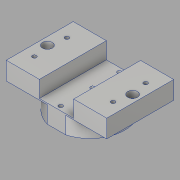
# Autodesk Inventor part: PocketNC_Vise_Backing_Plate
Saved by Autodesk Inventor 2017 (Build 210142000, 142)
## iProperties
Created: 2018-06-05
Part Number: PocketNC_Vise_Backing_Plate
Material: Aluminum 6061
Document SubType Name: Modeling
Designer: Jarrett
Density: 2.7 g/cm^3
Appearance: Aluminum - Flat
Author: Jarrett
Autodesk Inventor part; units mm, degrees
ref_plane "YZ Plane" through (0, 0, 0) normal (1, 0, 0) x (0, 1, 0)
ref_plane "XZ Plane" through (0, 0, 0) normal (0, 1, 0) x (-1, 0, 0)
ref_plane "XY Plane" through (0, 0, 0) normal (0, 0, 1) x (1, 0, 0)
sketch "Sketch1" plane through (0, 0, 0) normal (0, 1, 0) x (-1, 0, 0)
  line L0 (37.5, -25) -> (-37.5, -25) construction
  line L1 (-37.5, -25) -> (-37.5, 25) construction
  line L2 (-37.5, 25) -> (37.5, 25) construction
  line L3 (37.5, 25) -> (37.5, -25) construction
  arc A0 (6.8822, -25) -> (6.8822, 25) centre (0, 0) ccw
  arc A1 (-6.8822, 25) -> (-6.8822, -25) centre (0, 0) ccw
  line L4 (6.8822, -25) -> (-6.8822, -25)
  line L5 (-6.8822, 25) -> (6.8822, 25)
  dimension "d4" = 50
  dimension "d5" = 75
  constraints: 12 end point, 4 point on circle, 4 point on line, 2 centre point, 2 collinear, 1 coincident, 1 perpendicular, 1 vertical
  measures "d4" distance of L0.end L1.end
  measures "d5" distance of L1.end L2.end
extrude "Extrusion1" add sketch "Sketch1" along normal blind 12.65
sketch "Sketch2" plane through (0, 12.65, 0) normal (0, 1, 0) x (1, 0, 0)
  line L0 (-37.5, 25) -> (37.5, 25) construction
  line L1 (-37.5, -25) -> (-37.5, 25) construction
  line L2 (37.5, 25) -> (37.5, -25) construction
  line L3 (37.5, -25) -> (-37.5, -25) construction
  line L4 (-37.5, 25) -> (37.5, 25)
  line L5 (37.5, -25) -> (37.5, 25)
  line L6 (37.5, -25) -> (-37.5, -25)
  line L7 (-37.5, -25) -> (-37.5, 25)
  point P0 (0, 0)
  constraints: 8 end point, 2 collinear, 1 horizontal, 1 perpendicular
extrude "Extrusion2" add sketch "Sketch2" along normal blind 1
sketch "Sketch3" plane through (0, 13.65, 0) normal (0, 1, 0) x (1, 0, 0)
  line L0 (37.5, -25) -> (6.8822, -25) projected
  line L1 (12.8, -25) -> (12.8, 25)
  line L2 (12.8, 25) -> (37.5, 25)
  line L3 (37.5, -25) -> (37.5, 25) projected
  line L4 (37.5, 25) -> (37.5, -25)
  line L5 (37.5, -25) -> (12.8, -25)
  line L6 (-12.8, -25) -> (-12.8, 25)
  line L7 (-37.5, 25) -> (-37.5, -25) projected
  line L8 (-12.8, 25) -> (-37.5, 25)
  line L9 (-37.5, 25) -> (-37.5, -25)
  line L10 (-37.5, -25) -> (-12.8, -25)
  point P0 (0, 0)
  dimension "d12" = 25.6
  dimension "d13" = 24.7
  dimension "d14" = 24.7
  constraints: 16 end point, 4 perpendicular, 2 collinear, 2 point on line, 1 vertical
  measures "d12" distance between parallel lines of L1 L6
  measures "d13" distance of L6.end L7.start
  measures "d14" distance of L1.end L2.end
extrude "Extrusion3" add sketch "Sketch3" along normal blind 12.4 contours L10 L7 L8 L6
extrude "Extrusion4" add sketch "Sketch3" along normal blind 12.45 contours L0 L1 L2 L3
sketch "Sketch4" plane through (0, 13.65, 0) normal (0, 1, 0) x (1, 0, 0)
  circle A0 centre (0, 21.91) radius 1.5
  circle A1 centre (0, -21.91) radius 1.5
  circle A2 centre (0, 1.95) radius 1.5
  line L0 (12.8, 25) -> (12.8, -25) projected
  point P0 (0, 0)
  dimension "d21" = 3
  dimension "d23" = 3
  dimension "d25" = 3
  dimension "d26" = 21.91
  dimension "d27" = 23.86
  dimension "d28" = 21.91
  dimension "d29" = 12.8
  constraints: 3 centre point
  measures "d21" diameter of A0
  measures "d23" diameter of A1
  measures "d25" diameter of A2
  measures "d26" distance of point (0, 0) A0.centre
  measures "d27" distance of A1.centre A2.centre
  measures "d28" distance of point (0, 0) A1.centre
  measures "d29" distance from line of L0 A0.centre
extrude "Extrusion5" cut sketch "Sketch4" against normal blind 18.8
sketch "Sketch5" plane through (0, 26.05, 0) normal (0, 1, 0) x (1, 0, 0)
  circle A0 centre (-29.4, 12.15) radius 1.5
  circle A1 centre (-29.4, -12.15) radius 1.5
  circle A2 centre (-31.8, 0) radius 2.2
  line L0 (-37.5, 25) -> (-37.5, -25) projected
  circle A3 centre (29.4, 12.15) radius 1.5
  circle A4 centre (29.4, -12.15) radius 1.5
  circle A5 centre (31.8, 0) radius 2.2
  circle A6 centre (29.4, 12.15) radius 1.5
  circle A7 centre (29.4, -12.15) radius 1.5
  circle A8 centre (31.8, 0) radius 2.2
  point P0 (0, 0)
  dimension "d35" = 3
  dimension "d36" = 3
  dimension "d37" = 4.4
  dimension "d38" = 8.1
  dimension "d41" = 5.7
  constraints: 9 centre point
  measures "d35" diameter of A0
  measures "d36" diameter of A1
  measures "d37" diameter of A2
  measures "d38" distance from line of L0 A0.centre
  measures "d41" distance from line of L0 A2.centre
extrude "Extrusion6" cut sketch "Sketch5" along normal mid plane 35
sketch "Sketch7" plane through (0, 26.1, 0) normal (0, 1, 0) x (1, 0, 0)
  circle A0 centre (31.8, 0) radius 3.7
  point P0 (0, 0)
  dimension "d44" = 7.4
  constraints: 1 centre point, 1 coincident
  measures "d44" diameter of A0
extrude "Extrusion7" cut sketch "Sketch7" against normal blind 5
sketch "Sketch8" plane through (0, 26.05, 0) normal (0, 1, 0) x (1, 0, 0)
  circle A0 centre (-31.8, 0) radius 3.7
  point P0 (0, 0)
  dimension "d47" = 7.4
  constraints: 1 centre point, 1 coincident
  measures "d47" diameter of A0
extrude "Extrusion8" cut sketch "Sketch8" against normal blind 5
body "Solid1"
